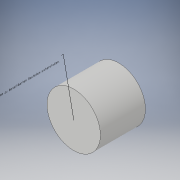
# Autodesk Inventor part: Gehäuse
Saved by Autodesk Inventor 2019 (Build 230136000, 136)
## iProperties
Created: 2022-03-18
Part Number: Gehäuse
Material: Generisch
Document SubType Name: Modeling
Designer: deka
Density: 1 g/cm^3
Appearance: Vorgabe
Title: E:\SynologyDrive\XMI_Schnittstelle\Daten\Blank_STEP_Inventor.stp
Author: dkac11
Sending System: Autodesk Inventor 2019
Preprocessor: ST-DEVELOPER v17
Autodesk Inventor part; units mm, degrees
ref_plane "YZ Plane" through (0, 0, 0) normal (1, 0, 0) x (0, 1, 0)
ref_plane "XZ Plane" through (0, 0, 0) normal (0, 1, 0) x (-1, 0, 0)
ref_plane "XY Plane" through (0, 0, 0) normal (0, 0, 1) x (1, 0, 0)
sketch "Skizze1" plane through (0, 0, 0) normal (0, 0, 1) x (1, 0, 0)
  circle A0 centre (0, 0) radius 14.8151
  constraints: 1 centre point, 1 coincident
extrude "Extrusion1" add sketch "Skizze1" along normal blind 25
